mipi hdmi gb (Autodesk Fusion 360 design; units mm, degrees)
Autodesk Fusion 360 part; units mm, degrees
sketch "Sketch1" plane through (0, 0, 0) normal (0, 1, 0) x (1, 0, 0) in component "atom"
  line L0 (3.30721, -13.488035) -> (4.10711, -14.291522)
  line L1 (4.10711, -14.291522) -> (4.813748, -14.277174)
  line L2 (4.813748, -14.277174) -> (4.824509, -14.359674)
  line L3 (4.824509, -14.359674) -> (5.003859, -14.370435)
  line L4 (5.003859, -14.370435) -> (5.000272, -14.521089)
  line L5 (5.000272, -14.521089) -> (5.118642, -14.617937)
  line L6 (5.118642, -14.617937) -> (7.012576, -14.646633)
  line L7 (7.012576, -14.646633) -> (7.116599, -14.539024)
  line L8 (7.116599, -14.539024) -> (7.105838, -14.391957)
  line L9 (7.105838, -14.391957) -> (7.281601, -14.395542)
  line L10 (7.281601, -14.395542) -> (7.278016, -14.284345)
  line L11 (7.278016, -14.284345) -> (7.64389, -14.28076)
  line L12 (7.64389, -14.28076) -> (8.027698, -14.657394)
  line L13 (8.027698, -14.657394) -> (8.067155, -17.849821)
  line L14 (8.067155, -17.849821) -> (7.981067, -17.925147)
  line L15 (7.981067, -17.925147) -> (7.98824, -18.520589)
  line L16 (7.98824, -18.520589) -> (8.461723, -18.520589)
  line L17 (8.461723, -18.520589) -> (8.461723, -18.714287)
  line L18 (8.461723, -18.714287) -> (10.057936, -18.714287)
  line L19 (10.057936, -18.714287) -> (10.057936, -18.53135)
  line L20 (10.057936, -18.53135) -> (10.578051, -18.53135)
  line L21 (10.578051, -18.53135) -> (10.922402, -18.190587)
  line L22 (10.922402, -18.190587) -> (10.958272, -18.183414)
  line L23 (10.958272, -18.183414) -> (10.969032, -18.699943)
  line L24 (10.969032, -18.699943) -> (11.959044, -18.699943)
  line L25 (11.959044, -18.699943) -> (12.464811, -18.520593)
  line L26 (12.464811, -18.520593) -> (14.92549, -18.520593)
  line L27 (14.92549, -18.520593) -> (14.903969, -18.043523)
  line L28 (14.903969, -18.043523) -> (15.17867, -17.778921)
  line L29 (15.17867, -17.778921) -> (15.226798, -16.318177)
  line L30 (15.226798, -16.318177) -> (15.343672, -16.164773)
  line L31 (15.343672, -16.164773) -> (16.896841, -16.164773)
  line L32 (16.896841, -16.164773) -> (17.033148, -16.319014)
  line L33 (17.033148, -16.319014) -> (17.039337, -18.100853)
  line L34 (17.039337, -18.100853) -> (17.346953, -18.401867)
  line L35 (17.346953, -18.401867) -> (17.596935, -18.644867)
  line L36 (17.596935, -18.644867) -> (17.66446, -18.654148)
  line L37 (17.66446, -18.654148) -> (19.40774, -18.654148)
  line L38 (19.40774, -18.654148) -> (19.40774, -18.24523)
  line L39 (19.40774, -18.24523) -> (19.544045, -18.083816)
  line L40 (19.544045, -18.083816) -> (20.846125, -18.083816)
  line L41 (20.846125, -18.083816) -> (20.986017, -18.349253)
  line L42 (20.986017, -18.349253) -> (21.387761, -18.349253)
  line L43 (21.387761, -18.349253) -> (21.387761, -18.525016)
  line L44 (21.387761, -18.525016) -> (21.172541, -18.525016)
  line L45 (21.172541, -18.525016) -> (21.172541, -18.722301)
  line L46 (21.172541, -18.722301) -> (23.206368, -18.722301)
  line L47 (23.206368, -18.722301) -> (23.206368, -18.564472)
  line L48 (23.206368, -18.564472) -> (23.052126, -18.564472)
  line L49 (23.052126, -18.564472) -> (23.052126, -18.342077)
  line L50 (23.052126, -18.342077) -> (23.504089, -18.342077)
  line L51 (23.504089, -18.342077) -> (23.647567, -18.112509)
  line L52 (23.647567, -18.112509) -> (23.672677, -18.062292)
  line L53 (23.672677, -18.062292) -> (27.210845, -18.025168)
  line L54 (27.210845, -18.025168) -> (29.221551, -17.335788)
  line L55 (29.221551, -17.335788) -> (29.336824, -17.124108)
  line L56 (29.336824, -17.124108) -> (29.351507, -3.590552)
  line L57 (29.351507, -3.590552) -> (3.26936, -3.584366)
  line L58 (3.26936, -3.584366) -> (3.30721, -13.488035)
  circle A0 centre (19.790975, -16.395454) radius 0.193272
  circle A1 centre (28.939667, -16.96424) radius 0.193272
  circle A2 centre (10.390977, -16.45527) radius 0.193272
  line L59 (26.297155, -14.694613) -> (28.413822, -14.694613)
  line L60 (28.413822, -14.694613) -> (28.413822, -17.075863)
  line L61 (28.413822, -17.075863) -> (26.297155, -17.075863)
  line L62 (26.297155, -17.075863) -> (26.297155, -14.694613)
  line L63 (3.274216, -3.589223) -> (29.366975, -3.589223)
  line L64 (29.366975, -3.589223) -> (29.366975, -18.705304)
  line L65 (29.366975, -18.705304) -> (3.274216, -18.705304)
  line L66 (3.274216, -18.705304) -> (3.274216, -3.589223)
  line L67 (1.570909, -1.43053) -> (31.570909, -1.43053)
  line L68 (31.570909, -1.43053) -> (31.570909, -19.93053)
  line L69 (31.570909, -19.93053) -> (1.570909, -19.93053)
  line L70 (1.570909, -19.93053) -> (1.570909, -1.43053)
  point P0 (19.984248, -16.395454)
  point P1 (29.132939, -16.96424)
  point P2 (10.584249, -16.45527)
  dimension "d9" = 30
  dimension "d10" = 18.5
  constraint horizontal L67
  constraint vertical L68
  constraint horizontal L69
  constraint vertical L70
sketch "Sketch1 (2)" plane through (0, 0, 0) normal (0, 1, 0) x (1, 0, 0) in component "mipi hdmi"
  line L0 (7.54697, -5.345109) -> (22.892803, -5.345109)
  arc A0 (22.892803, -5.345109) -> (23.686553, -6.138859) centre (22.892803, -6.138859) cw
  line L1 (23.686553, -6.138859) -> (23.686553, -21.749276)
  arc A1 (23.686553, -21.749276) -> (22.892803, -22.543026) centre (22.892803, -21.749276) cw
  line L2 (22.892803, -22.543026) -> (7.54697, -22.543026)
  arc A2 (7.54697, -22.543026) -> (6.75322, -21.749276) centre (7.54697, -21.749276) cw
  line L3 (6.75322, -21.749276) -> (6.75322, -6.138859)
  arc A3 (6.75322, -6.138859) -> (7.54697, -5.345109) centre (7.54697, -6.138859) cw
  line L4 (6.740323, -9.039008) -> (8.06324, -9.039008)
  line L5 (8.06324, -9.039008) -> (8.06324, -18.299425)
  line L6 (8.06324, -18.299425) -> (6.740323, -18.299425)
  line L7 (6.740323, -18.299425) -> (6.740323, -9.039008)
  line L8 (20.852543, -12.125257) -> (24.027543, -12.125257)
  line L9 (24.027543, -12.125257) -> (24.027543, -16.094007)
  line L10 (24.027543, -16.094007) -> (20.852543, -16.094007)
  line L11 (20.852543, -16.094007) -> (20.852543, -12.125257)
  line L12 (22.121371, -18.500028) -> (23.973455, -18.500028)
  line L13 (23.973455, -18.500028) -> (23.973455, -20.616694)
  line L14 (23.973455, -20.616694) -> (22.121371, -20.616694)
  line L15 (22.121371, -20.616694) -> (22.121371, -18.500028)
  circle A4 centre (9.797923, -6.222293) radius 0.330729
  circle A5 centre (9.797923, -21.650874) radius 0.330729
  circle A6 centre (22.776619, -6.222293) radius 0.330729
  point P0 (10.128652, -6.222293)
  point P1 (10.128652, -21.650874)
  point P2 (23.107348, -6.222293)
sketch "Sketch1 (3)" plane through (0, 0, 0) normal (0, 1, 0) x (1, 0, 0) in component "mipi adapter"
  line L0 (2.51375, -2.224515) -> (10.284563, -2.224515)
  line L1 (10.284563, -2.224515) -> (10.284563, -20.930556)
  line L2 (10.284563, -20.930556) -> (2.51375, -20.930556)
  line L3 (2.51375, -20.930556) -> (2.51375, -2.224515)
  circle A0 centre (2.873279, -2.57524) radius 0.178628
  circle A1 centre (2.873279, -20.493071) radius 0.178628
  circle A2 centre (9.951067, -2.57524) radius 0.178628
  line L4 (2.530814, -6.79048) -> (3.853731, -6.79048)
  line L5 (3.853731, -6.79048) -> (3.853731, -16.050897)
  line L6 (3.853731, -16.050897) -> (2.530814, -16.050897)
  line L7 (2.530814, -16.050897) -> (2.530814, -6.79048)
  line L8 (7.217884, -2.713434) -> (9.585151, -2.713434)
  line L9 (9.585151, -2.713434) -> (9.585151, -3.374139)
  line L10 (9.585151, -3.374139) -> (7.217884, -3.374139)
  line L11 (7.217884, -3.374139) -> (7.217884, -2.713434)
  line L12 (7.217884, -19.72888) -> (9.585151, -19.72888)
  line L13 (9.585151, -19.72888) -> (9.585151, -20.389585)
  line L14 (9.585151, -20.389585) -> (7.217884, -20.389585)
  line L15 (7.217884, -20.389585) -> (7.217884, -19.72888)
  point P0 (3.051906, -2.57524)
  point P1 (3.051906, -20.493071)
  point P2 (10.129694, -2.57524)
extrude "Extrude1" add sketch "Sketch1" along normal blind 3 contours L0 L1 L2 L3 L4 L5 L6 L7 L8 L9 L10 L11 L12 L13 L14 L15 L16 L17 L19 L20 L21 L22 L23 L24 L25 L26 L27 L28 L29 L30 L31 L32 L33 L34 L35 L36 L37 L38 L39 L40 L41 L42 L43 L44 L45 L47 L48 L49 L50 L51 L52 L53 L54 L55 L56 L58 L63 L65 L66 picked at (16.507521, -7.781516) makes body 1 in component "atom"
extrude "Extrude2" add sketch "Sketch1 (3)" along normal blind 3 separate body contours L0 L1 L2 L3 picked at (7.674678, -13.051305) sketch seen with x (1, 0, 0) y (0, 1, 0) z (0, 0, 1) at (-9, 0, 15) makes body 2 in component "atom"
extrude "Extrude3" add sketch "Sketch1 (2)" along normal blind 3 separate body contours L0 A0 L1 A1 L2 A2 L3 A3 L4 L5 L6 L8 L10 L11 L12 L14 L15 picked at (12.326341, -13.154563) sketch seen with x (1, 0, 0) y (0, 1, 0) z (0, 0, 1) at (-1, 0, 15) makes body 3 in component "atom"
copy_body "CutPasteBodies1" bodies 2 body 2 seen with x (1, 0, 0) y (0, 1, 0) z (0, 0, 1) at (9, 0, -15) removing the originals makes body 4 in component "mipi adapter"
copy_body "CutPasteBodies1'" bodies 3 body 3 seen with x (1, 0, 0) y (0, 1, 0) z (0, 0, 1) at (1, 0, -15) removing the originals makes body 5 in component "mipi hdmi"
extrude "Extrude4" cut sketch "Sketch1" along normal blind 2.5 contours L0 L1 L2 L3 L4 L5 L6 L7 L8 L9 L10 L11 L12 L13 L14 L15 L16 L17 L19 L20 L21 L22 L23 L24 L25 L26 L27 L28 L29 L30 L31 L32 L33 L34 L35 L36 L37 L38 L39 L40 L41 L42 L43 L44 L45 L47 L48 L49 L50 L51 L52 L53 L54 L55 L56 L58 L63 L65 L66 picked at (16.507521, -7.781516) bodies 1 in component "atom"
extrude "Extrude5" add sketch "Sketch1" along normal blind 3 contours L0 L1 L2 L3 L4 L5 L6 L7 L8 L9 L10 L11 L12 L13 L14 L15 L16 L17 L58 L65 L66 | L47 L48 L49 L50 L51 L52 L53 L54 L55 L56 L57 L63 L64 L65 | L19 L20 L21 L22 L23 L24 L25 L26 L27 L28 L29 L30 L31 L32 L33 L34 L35 L36 L37 L38 L39 L40 L41 L42 L43 L44 L45 L65 | L67 L68 L69 L70 picked at (5.457975, -17.082796) picked at (28.59979, -18.022087) picked at (16.417051, -17.399596) picked at (18.963296, -2.150094) bodies 1 in component "atom"
extrude "Extrude6" add sketch "Sketch1" along normal blind 3 contours A2 picked at (10.337747, -16.418979) bodies 1 in component "atom"
extrude "Extrude7" add sketch "Sketch1" along normal blind 3 contours A0 picked at (19.838202, -16.439274) bodies 1 in component "atom"
extrude "Extrude8" add sketch "Sketch1" along normal blind 3 contours A1 picked at (28.986893, -17.008059) bodies 1 in component "atom"
extrude "Extrude9" add sketch "Sketch1" along normal blind 3 contours L59 L60 L61 L62 picked at (27.002711, -15.488363) bodies 1 in component "atom"
component "atom" placed x (1, 0, 0) y (0, 1, 0) z (0, 0, 1) at (3.3, 0, -15.5)
component "mipi hdmi" placed x (1, 0, 0) y (0, 1, 0) z (0, 0, 1) at (9, 3, -17)
component "mipi adapter" placed x (1, 0, 0) y (0, 1, 0) z (0, 0, 1) at (4, 3, -14)
